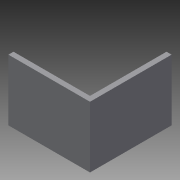
# Autodesk Inventor part: L-Frame Small
Saved by Autodesk Inventor 2015 (Build 190159000, 159)
## iProperties
Created: 2015-01-10
Part Number: L-Frame Small
Material: Generic
Document SubType Name: Modeling
Designer: Chandler Willoughby
Density: 1 g/cm^3
Appearance: Default
Author: Chandler Willoughby
Autodesk Inventor part; units mm, degrees
ref_plane "YZ Plane" through (0, 0, 0) normal (1, 0, 0) x (0, 1, 0)
ref_plane "XZ Plane" through (0, 0, 0) normal (0, 1, 0) x (-1, 0, 0)
ref_plane "XY Plane" through (0, 0, 0) normal (0, 0, 1) x (1, 0, 0)
sketch "Sketch1" plane through (0, 0, 0) normal (0, 1, 0) x (-1, 0, 0)
  line L0 (0, 0) -> (50.8, 0)
  line L1 (50.8, 0) -> (50.8, -3.175)
  line L2 (50.8, -3.175) -> (3.175, -3.175)
  line L3 (3.175, -3.175) -> (3.175, -50.8)
  line L4 (3.175, -50.8) -> (0, -50.8)
  line L5 (0, -50.8) -> (0, 0)
  dimension "d0" = 50.8
  dimension "d1" = 3.175
  dimension "d2" = 47.625
  dimension "d3" = 47.625
  constraints: 12 end point, 5 perpendicular, 1 horizontal
  measures "d0" distance of L0.start L0.end
  measures "d1" distance of L0.end L1.end
  measures "d2" distance of L1.end L2.end
  measures "d3" distance of L2.end L3.end
extrude "Extrusion1" add sketch "Sketch1" along normal blind 38.1
body "Solid1"
